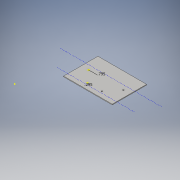
# Autodesk Inventor part: track side panel V1.1
Saved by Autodesk Inventor 2016 (Build 200138000, 138)
## iProperties
Created: 2015-10-10
Part Number: track side panel V1.1
Material: Generic
Document SubType Name: Modeling
Designer: Delta
Density: 1 g/cm^3
Appearance: Default
Author: Delta
Autodesk Inventor part; units mm, degrees
ref_plane "YZ Plane" through (0, 0, 0) normal (1, 0, 0) x (0, 1, 0)
ref_plane "XZ Plane" through (0, 0, 0) normal (0, 1, 0) x (-1, 0, 0)
ref_plane "XY Plane" through (0, 0, 0) normal (0, 0, 1) x (1, 0, 0)
sketch "Sketch1" plane through (0, 0, 0) normal (0, 1, 0) x (-1, 0, 0)
  line L0 (-77.6185, -139.5068) -> (-293.5185, -139.5068)
  line L1 (-293.5185, -139.5068) -> (-293.5185, -291.9068)
  line L2 (-293.5185, -291.9068) -> (-77.6185, -291.9068)
  line L3 (-77.6185, -291.9068) -> (-77.6185, -139.5068)
  point P0 (0, 0)
  dimension "d0" = 215.9
  dimension "d1" = 152.4
  constraints: 8 end point, 2 parallel, 1 horizontal, 1 perpendicular
  measures "d0" distance of L2.end L1.end
  measures "d1" distance of L1.end L0.end
extrude "Extrusion1" add sketch "Sketch1" along normal blind 3.175
sketch "Sketch2" plane through (0, 3.175, 0) normal (0, 1, 0) x (1, 0, 0)
  line L0 (77.6185, 291.9068) -> (77.6185, 139.5068) projected
  line L1 (77.6185, 139.5068) -> (293.5185, 139.5068) projected
  line L2 (293.5185, 139.5068) -> (293.5185, 291.9068) projected
  line L3 (293.5185, 291.9068) -> (77.6185, 291.9068) projected
  point P0 (0, 0)
  point P1 (156.9685, 165.5068)
  point P2 (108.9685, 218.5068)
  point P3 (263.9685, 218.5068)
  point P4 (221.9685, 165.5068)
  dimension "d4" = 144.35
  dimension "d5" = 26
  dimension "d7" = 79
  dimension "d19" = 31.35
  dimension "d20" = 79
  dimension "d21" = 26
  dimension "d22" = 79.35
  dimension "d23" = 186.35
  measures "d4" distance from line of L0 point (221.968, 165.507)
  measures "d5" distance from line of L1 point (221.968, 165.507)
  measures "d7" distance from line of L1 point (263.968, 218.507)
  measures "d19" distance from line of L0 point (108.968, 218.507)
  measures "d20" distance from line of L1 point (108.968, 218.507)
  measures "d21" distance from line of L1 point (156.968, 165.507)
  measures "d22" distance from line of L0 point (156.968, 165.507)
  measures "d23" distance from line of L0 point (263.968, 218.507)
hole "Hole1" at (156.9685, 3.175, -165.5068) at (108.9685, 3.175, -218.5068) at (263.9685, 3.175, -218.5068) at (221.9685, 3.175, -165.5068) direction (0, -1, 0) diameter 6 end through all
sketch "Sketch5" plane through (0, 3.175, 0) normal (0, 1, 0) x (1, 0, 0)
  line L0 (27.3395, 158.0068) -> (376.3264, 158.0068) construction
  line L1 (-38.6381, 238.7068) -> (415.1027, 238.7068) construction
  circle A0 centre (156.9685, 165.5068) radius 3 projected
  circle A1 centre (108.9685, 218.5068) radius 3 projected
  point P0 (0, 0)
  dimension "d45" = 7.5
  dimension "d46" = 20.2
  constraints: 4 end point, 2 horizontal
  measures "d45" distance from line of L0 A0.centre
  measures "d46" distance from line of L1 A1.centre
body "Solid1"
